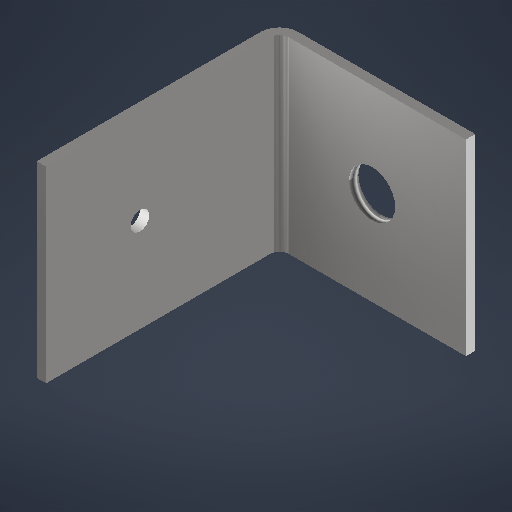
# Autodesk Inventor part: Pressure plate tab_L
Saved by Autodesk Inventor 2026.3 (Build 303398000, 398)
## iProperties
Created: 2026-08-04
Part Number: Pressure plate tab_L
Material: Generic
Document SubType Name: Sheet Metal
Designer: matot
Density: 1 g/cm^3
Sheet Metal Rule: Default_mm
Appearance: Default
Author: matot
Autodesk Inventor part; units mm, degrees
ref_plane "YZ Plane" through (0, 0, 0) normal (1, 0, 0) x (0, 1, 0)
ref_plane "XZ Plane" through (0, 0, 0) normal (0, 1, 0) x (-1, 0, 0)
ref_plane "XY Plane" through (0, 0, 0) normal (0, 0, 1) x (1, 0, 0)
sketch "Sketch1" plane through (0, 0, 0) normal (1, 0, 0) x (0, 1, 0)
  line L0 (12.963, 18.5185) -> (-7.037, 18.5185)
  line L1 (-7.037, 18.5185) -> (-7.037, -31.4815)
  line L2 (-7.037, -31.4815) -> (12.963, -31.4815)
  line L3 (12.963, -31.4815) -> (12.963, 18.5185)
  point P0 (0, 0)
  dimension "d0" = 50
  dimension "d1" = 20
  measures "d0" distance of L2.end L0.start
  measures "d1" distance of L1.end L2.end
extrude "Plate1" add sketch "Sketch1" along normal blind 1
sketch "Sketch2" plane through (1, 0, 0) normal (1, 0, 0) x (0, 0, -1)
  line L0 (31.4815, 12.963) -> (-18.5185, 12.963) projected
  line L1 (6.4815, 12.963) -> (6.4815, -7.037)
  line L2 (31.4815, -7.037) -> (-18.5185, -7.037) projected
  line L3 (-18.5185, -7.037) -> (-18.5185, 12.963) projected
  point P0 (0, 0)
  dimension "d3" = 20
  dimension "d4" = 25
  constraints: 2 end point, 1 midpoint, 1 perpendicular, 1 vertical
  measures "d3" distance of L1.start L1.end
  measures "d4" distance between parallel lines of L3 L1
fold "Fold1" angle 90 bend radius 1 thickness 1 k factor 0.44 line from (1, 12.963, -6.4815) to (1, -7.037, -6.4815) line at bend centre moving side (0, 0, -1) folds toward (1, 0, 0)
sketch "Sketch3" plane through (25.869, 12.963, -7.3505) normal (0, 0, -1) x (-1, 0, 0)
  line L0 (0, -20) -> (0, 0) projected
  line L1 (23.869, -20) -> (0, -20) projected
  point P0 (25.869, -12.963)
  point P1 (15, -10)
  point P2 (0, -10)
  dimension "d11" = 15
  dimension "d12" = 10
  constraints: 1 midpoint
  measures "d11" distance of point (0, -10) point (15, -10)
  measures "d12" distance from line of L1 point (15, -10)
hole "Hole1" at (10.869, 2.963, -7.3505) direction (0, 0, 1) diameter 4.917 depth 17.1 tip angle 118 thread size "M6x1" class "6H" standard "ISO Metric profile"
sketch "Sketch4" plane through (1, 0, 0) normal (1, 0, 0) x (0, 0, -1)
  line L0 (-18.5185, -7.037) -> (-18.5185, 12.963) projected
  line L1 (-18.5185, 12.963) -> (5.3505, 12.963) projected
  point P0 (0, 0)
  point P1 (-8.5185, 2.963)
  point P2 (-18.5185, 2.963)
  dimension "d20" = 10
  dimension "d21" = 10
  constraints: 1 midpoint
  measures "d20" distance of point (-8.519, 2.963) point (-18.519, 2.963)
  measures "d21" distance from line of point (-8.519, 2.963) L1
hole "Hole2" at (1, 2.963, 8.5185) direction (-1, 0, 0) diameter 2 end through all
sketch "Sketch5" plane through (2, -7.037, -6.3505) normal (0, 0, 1) x (1, 0, 0)
  line L0 (0, 20) -> (23.869, 20) projected
  line L1 (18.869, 20) -> (18.869, 0)
  line L2 (23.869, 0) -> (0, 0) projected
  line L3 (23.869, 20) -> (23.869, 0) projected
  point P0 (-2, 7.037)
  dimension "d29" = 5
  constraints: 2 end point, 2 point on line, 1 vertical
  measures "d29" distance between parallel lines of L3 L1
extrude "Cut1" cut sketch "Sketch5" against normal through all
equation "\"d2\" = Thickness"
equation "\"d5\" = BendReliefWidth"
equation "\"d6\" = BendReliefDepth"
equation "\"d7\" = MinimumRemnant"
equation "\"d8\" = TransitionRadius"
equation "\"d10\" = BendRadius"
equation "\"d27\" = Thickness"
equation "\"d30\" = Thickness"
equation "\"BendRadius\" = Thickness"
equation "\"BendReliefWidth\" = Thickness"
equation "\"BendReliefDepth\" = 0.5 * Thickness"
equation "\"CornerReliefSize\" = 4 * Thickness"
equation "\"MinimumRemnant\" = 2 * Thickness"
equation "\"TransitionRadius\" = BendRadius"
equation "\"JacobiRadiusSize\" = BendRadius"
equation "\"GapSize\" = Thickness"
equation "\"Thickness\" = 1"
body "Solid1"
